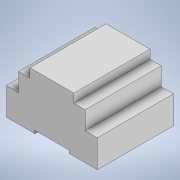
# Autodesk Inventor part: Supply
Saved by Autodesk Inventor 2020 (Build 240168000, 168)
## iProperties
Created: 2019-12-11
Part Number: Supply
Material: Generic
Document SubType Name: Modeling
Designer: nicoc
Density: 1 g/cm^3
Appearance: Default
Author: nicoc
Autodesk Inventor part; units mm, degrees
ref_plane "YZ Plane" through (0, 0, 0) normal (1, 0, 0) x (0, 1, 0)
ref_plane "XZ Plane" through (0, 0, 0) normal (0, 1, 0) x (-1, 0, 0)
ref_plane "XY Plane" through (0, 0, 0) normal (0, 0, 1) x (1, 0, 0)
sketch "Sketch1" plane through (0, 0, 0) normal (0, 1, 0) x (-1, 0, 0)
  line L0 (0, 0) -> (93, 0)
  line L1 (93, 0) -> (93, -78)
  line L2 (93, -78) -> (0, -78)
  line L3 (0, -78) -> (0, 0)
  dimension "d0" = 78
  dimension "d1" = 93
  constraints: 8 end point, 2 parallel, 1 horizontal, 1 perpendicular
  measures "d0" distance between parallel lines of L2 L0
  measures "d1" distance between parallel lines of L1 L3
extrude "Extrusion1" add sketch "Sketch1" along normal blind 56
sketch "Sketch2" plane through (0, 0, 0) normal (0, -1, 0) x (1, 0, 0)
  line L0 (-93, 0) -> (0, 0) projected
  line L1 (0, -78) -> (-93, -78) projected
  line L2 (-29, 0) -> (-64, 0)
  line L3 (-64, 0) -> (-64, -78)
  line L4 (-64, -78) -> (-29, -78)
  line L5 (-29, -78) -> (-29, 0)
  line L6 (-93, -78) -> (-93, 0) projected
  dimension "d4" = 29
  dimension "d5" = 35
  constraints: 8 end point, 2 parallel, 2 point on line, 1 horizontal, 1 perpendicular
  measures "d4" distance between parallel lines of L3 L6
  measures "d5" distance between parallel lines of L5 L3
extrude "Extrusion2" cut sketch "Sketch2" against normal blind 3 contours L0 L5 L1 L3
sketch "Sketch3" plane through (0, 56, 0) normal (0, 1, 0) x (1, 0, 0)
  line L0 (0, 78) -> (-29, 78) projected
  line L1 (0, 0) -> (-12.5, 0)
  line L2 (-12.5, 0) -> (-12.5, 78)
  line L3 (-12.5, 78) -> (0, 78)
  line L4 (0, 78) -> (0, 0)
  line L5 (-93, 0) -> (-64, 0) projected
  line L6 (-93, 0) -> (-80.5, 0)
  line L7 (-80.5, 0) -> (-80.5, 78)
  line L8 (-80.5, 78) -> (-93, 78)
  line L9 (-93, 78) -> (-93, 0)
  dimension "d8" = 12.5
  dimension "d9" = 12.5
  constraints: 16 end point, 4 parallel, 2 horizontal, 2 perpendicular, 1 point on line
  measures "d8" distance between parallel lines of L2 L4
  measures "d9" distance between parallel lines of L9 L7
extrude "Extrusion3" cut sketch "Sketch3" against normal blind 27.6
sketch "Sketch4" plane through (0, 56, 0) normal (0, 1, 0) x (1, 0, 0)
  line L0 (-80.5, 0) -> (-12.5, 0) projected
  line L1 (-12.5, 78) -> (-80.5, 78) projected
  line L2 (-12.5, 0) -> (-24, 0)
  line L3 (-24, 0) -> (-24, 78)
  line L4 (-24, 78) -> (-12.5, 78)
  line L5 (-12.5, 78) -> (-12.5, 0)
  line L6 (-80.5, 0) -> (-69, 0)
  line L7 (-69, 0) -> (-69, 78)
  line L8 (-69, 78) -> (-80.5, 78)
  line L9 (-80.5, 78) -> (-80.5, 0)
  point P0 (0, 0)
  dimension "d12" = 11.5
  dimension "d13" = 11.5
  constraints: 16 end point, 4 parallel, 2 horizontal, 2 perpendicular, 2 point on line
  measures "d12" distance between parallel lines of L3 L5
  measures "d13" distance between parallel lines of L9 L7
extrude "Extrusion4" cut sketch "Sketch4" against normal blind 9 contours L9 L1 L7 L0 | L3 L1 L5 L0
body "Solid1"
